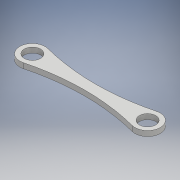
# Autodesk Inventor part: Arm 15X - actuator linkage
Saved by Autodesk Inventor 2017 (Build 210142000, 142)
## iProperties
Created: 2016-03-31
Part Number: Arm 15X - actuator linkage
Material: Generic
Document SubType Name: Modeling
Designer: alist
Density: 1 g/cm^3
Appearance: Default
Author: alist
## iProperties of the stored document Arm - actuator linkage_3DPrint.ipt
Created: 2017-01-15
Part Number: Arm - actuator linkage_3DPrint
Material: Generic
Document SubType Name: Modeling
Designer: Alistair
Density: 1 g/cm^3
Appearance: Default
Author: Alistair
Autodesk Inventor part; units mm, degrees
ref_plane "YZ Plane" through (0, 0, 0) normal (1, 0, 0) x (0, 1, 0)
ref_plane "XZ Plane" through (0, 0, 0) normal (0, 1, 0) x (-1, 0, 0)
ref_plane "XY Plane" through (0, 0, 0) normal (0, 0, 1) x (1, 0, 0)
sketch "Sketch1" plane through (0, 0, 0) normal (0, 0, 1) x (1, 0, 0)
  circle A0 centre (-77.5, 0) radius 11
  circle A1 centre (77.5, 0) radius 11
  arc A2 (-73.2027, 16.4479) -> (-73.2027, -16.4479) centre (-77.5, 0) ccw
  arc A3 (73.2027, -16.4479) -> (73.2027, 16.4479) centre (77.5, 0) ccw
  line L0 (-108.3592, 0) -> (107.2374, 0)
  arc A4 (-73.2027, 16.4479) -> (73.2027, 16.4479) centre (0, 296.6321) ccw
  arc A5 (73.2027, -16.4479) -> (-73.2027, -16.4479) centre (0, -296.6321) ccw
  point P0 (0, 0)
  dimension "d0" = 22
  dimension "d1" = 22
  dimension "d2" = 155
  dimension "d3" = 77.5
  dimension "d4" = 6
  dimension "d5" = 6
  constraints: 8 point on circle, 6 centre point, 3 point on line, 3 symmetric about line, 2 end point, 2 tangent, 1 horizontal, 1 other
  measures "d0" diameter of A0
  measures "d1" diameter of A1
  measures "d2" distance of A1.centre A0.centre
  measures "d3" distance of A1.centre point (0, 0)
  measures "d4" radial gap between concentric circles of A0 A2
  measures "d5" radial gap between concentric circles of A1 A3
extrude "Extrusion1" add sketch "Sketch1" along normal blind 7 contours L0 A1 A3 A5 A2 A0 | A0 L0 A2 A4 A3 A1
equation "\"d3\" = 0.5 * d2"
body "Solid1"
